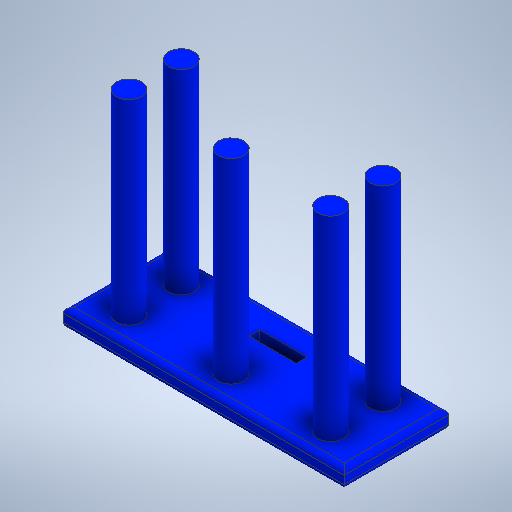
# Autodesk Inventor part: BluetoothBase
Saved by Autodesk Inventor 2025.2 (Build 292293000, 293)
## iProperties
Created: 2025-05-19
Part Number: BluetoothBase
Material: Generic
Document SubType Name: Modeling
Designer: User
Density: 1 g/cm^3
Appearance: Default
Author: User
Autodesk Inventor part; units mm, degrees
ref_plane "YZ Plane" through (0, 0, 0) normal (1, 0, 0) x (0, 1, 0)
ref_plane "XZ Plane" through (0, 0, 0) normal (0, 1, 0) x (-1, 0, 0)
ref_plane "XY Plane" through (0, 0, 0) normal (0, 0, 1) x (1, 0, 0)
sketch "Sketch1" plane through (0, 0, 0) normal (0, 1, 0) x (-1, 0, 0)
  circle A0 centre (0, 19.5421) radius 4.775
  circle A1 centre (-37.22, 0) radius 4.775
  circle A2 centre (38.1926, 0) radius 4.775
  circle A3 centre (38.1926, 19.5421) radius 4.775
  circle A4 centre (-37.22, 19.5421) radius 4.775
  line L0 (52.9676, 0) -> (52.9676, -4.775)
  line L1 (52.9676, -9.775) -> (-51.995, -9.775)
  line L2 (-51.995, -9.775) -> (-51.995, 24.3171)
  line L3 (-51.995, 24.3171) -> (-51.995, 29.3171)
  line L4 (-51.995, 29.3171) -> (52.9676, 29.3171)
  line L5 (52.9676, 29.3171) -> (52.9676, -9.775)
  line L6 (-8.8, 0) -> (8.8, 0)
  line L7 (8.8, 0) -> (8.8, 3.95)
  line L8 (8.8, 3.95) -> (-8.8, 3.95)
  line L9 (-8.8, 3.95) -> (-8.8, 0)
  point P0 (0, 0)
  point P1 (0, 0)
  dimension "d6" = 9.55
  dimension "d8" = 9.55
  dimension "d10" = 9.55
  dimension "d11" = 9.55
  dimension "d12" = 9.55
  dimension "d24" = 5
  dimension "d26" = 17.6
  dimension "d27" = 3.95
  constraints: 20 end point, 5 centre point, 5 perpendicular, 2 point on line, 2 vertical, 1 horizontal, 4 other
  measures "d6" diameter of A0
  measures "d8" diameter of A1
  measures "d10" diameter of A2
  measures "d11" diameter of A3
  measures "d12" diameter of A4
  measures "d24" distance of L2.end L3.end
  measures "d26" distance of L6.start L6.end
  measures "d27" distance of L6.end L7.end
extrude "Extrusion1" add sketch "Sketch1" along normal blind 7
extrude "Extrusion2" add sketch "Sketch1" along normal blind 80 contours A2 | A3
extrude "Extrusion3" add sketch "Sketch1" along normal blind 80 contours A1
extrude "Extrusion4" add sketch "Sketch1" along normal blind 80 contours A4
extrude "Extrusion5" add sketch "Sketch1" along normal blind 80 contours A0
fillet "Fillet1" radius 2 3 edges at (51.995, 7, 9.771) (-0.4863, 7, -9.775) (-0.4863, 7, 29.3171)
fillet "Fillet2" radius 2 3 edges at (-0.4863, 0, 29.3171) (-0.4863, 0, -9.775) (51.995, 0, 9.771)
body "Solid1"
